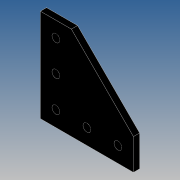
# Autodesk Inventor part: LPlate
Saved by Autodesk Inventor 2021 (Build 250183000, 183)
## iProperties
Created: 2021-02-20
Part Number: LPlate
Material: Aluminio 6061
Document SubType Name: Modeling
Designer: sddj_
Density: 2.7 g/cm^3
Appearance: Anodizado - Negro
Author: sddj_
Autodesk Inventor part; units mm, degrees
ref_plane "YZ Plane" through (0, 0, 0) normal (1, 0, 0) x (0, 1, 0)
ref_plane "XZ Plane" through (0, 0, 0) normal (0, 1, 0) x (-1, 0, 0)
ref_plane "XY Plane" through (0, 0, 0) normal (0, 0, 1) x (1, 0, 0)
sketch "Boceto1" plane through (0, 0, 0) normal (0, 0, 1) x (1, 0, 0)
  line L0 (190.1282, 320.5488) -> (475.893, 320.5488) construction
  line L1 (475.893, 320.5488) -> (475.893, 34.784) construction
  line L2 (475.893, 34.784) -> (190.1282, 34.784) construction
  line L3 (190.1282, 34.784) -> (190.1282, 320.5488) construction
  line L4 (0, 0) -> (0, 60)
  line L5 (0, 0) -> (60, 0)
  line L6 (60, 0) -> (60, 20)
  line L7 (60, 20) -> (20, 60)
  line L8 (20, 60) -> (0, 60)
  circle A0 centre (10, 50) radius 2.5
  circle A1 centre (10, 30) radius 2.5
  circle A2 centre (10, 10) radius 2.5
  circle A3 centre (30, 10) radius 2.5
  circle A4 centre (50, 10) radius 2.5
  point P0 (0, 30)
  point P1 (30, 0)
  dimension "d3" = 60
  dimension "d4" = 60
  dimension "d5" = 20
  dimension "d6" = 20
  dimension "d7" = 5
  dimension "d10" = 20
  dimension "d19" = 20
  constraints: 10 end point, 5 centre point, 2 horizontal, 2 midpoint, 2 vertical, 1 horizontal alignment, 1 parallel, 1 perpendicular, 1 vertical alignment, 10 other
  measures "d3" distance of L4.start L4.end
  measures "d4" distance of L4.start L5.end
  measures "d5" distance of L5.end L6.end
  measures "d6" distance of L7.end L4.end
  measures "d7" diameter of A0
  measures "d10" distance of A0.centre A1.centre
  measures "d19" distance of A2.centre A3.centre
extrude "Extrusión1" add sketch "Boceto1" along normal blind 4
